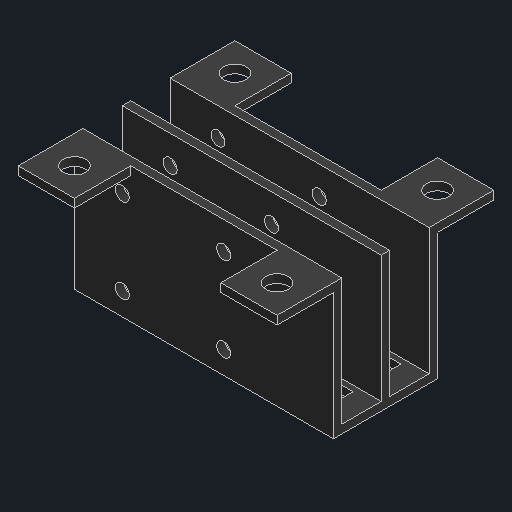
# Autodesk Inventor part: convertor_base
Saved by Autodesk Inventor 2026.1 (Build 301233020, 233B)
## iProperties
Created: 2025-11-26
Part Number: convertor_base
Material: 고무, 검은색
Document SubType Name: Modeling
Designer: jaewook
Density: 0.93 g/cm^3
Appearance: 고무 - 검은색
Author: jaewook
Autodesk Inventor part; units mm, degrees
ref_plane "YZ Plane" through (0, 0, 0) normal (1, 0, 0) x (0, 1, 0)
ref_plane "XZ Plane" through (0, 0, 0) normal (0, 1, 0) x (-1, 0, 0)
ref_plane "XY Plane" through (0, 0, 0) normal (0, 0, 1) x (1, 0, 0)
sketch "스케치1" plane through (0, 0, 0) normal (1, 0, 0) x (0, 1, 0)
  line L0 (12, -9.25) -> (-12, -9.25)
  line L1 (-12, -9.25) -> (-12, 9.25)
  line L2 (-12, 9.25) -> (12, 9.25)
  line L3 (12, 9.25) -> (12, -9.25)
  line L4 (12, -9.25) -> (-12, 9.25) construction
  line L5 (-12, -9.25) -> (12, 9.25) construction
  line L6 (12, 7.75) -> (-10.5, 7.75)
  line L7 (-10.5, 7.75) -> (-10.5, 0.75)
  line L8 (-10.5, 0.75) -> (12, 0.75)
  line L9 (12, 0.75) -> (12, 7.75)
  line L10 (-10.5, -7.75) -> (12, -7.75)
  line L11 (-10.5, -0.75) -> (-10.5, -7.75)
  line L12 (12, -0.75) -> (-10.5, -0.75)
  line L13 (12, 9.25) -> (13.5, 9.25)
  line L14 (13.5, 9.25) -> (13.5, -9.25)
  line L15 (13.5, -9.25) -> (12, -9.25)
  line L16 (12, -9.25) -> (12, 9.25)
  point P0 (0, 0)
  point P1 (12, -7.75)
  point P2 (12, -0.75)
  point P3 (-10, 7.75)
  point P4 (-10, -7.75)
  point P5 (-10, 0.75)
  point P6 (-10, -0.75)
  point P7 (-10, -0.75)
  point P8 (-10, -7.75)
  point P9 (12, 7.75)
  point P10 (12, -7.75)
  dimension "d0" = 24
  dimension "d1" = 18.5
  dimension "d2" = 22.5
  dimension "d3" = 7
  dimension "d4" = 1.5
  dimension "d7" = 8.5
  dimension "d18" = 1.5
  constraints: 34 end point, 6 parallel, 3 horizontal, 3 perpendicular, 2 midpoint, 1 collinear, 1 point on line, 1 vertical, 7 other
  measures "d0" distance of L1.end L2.end
  measures "d1" distance of L0.end L1.end
  measures "d2" distance of L8.end L7.end
  measures "d3" distance of L7.end L6.end
  measures "d4" distance between parallel lines of L2 L6
  measures "d7" distance of L7.end L10.start
  measures "d18" distance of L14.end L15.end
extrude "돌출1" add sketch "스케치1" against normal blind 45 contours L0 L1 L2 L3 L6 L7 L8 L12 L11 L10
sketch "스케치2" plane through (0, 0, 0) normal (1, 0, 0) x (0, 0, -1)
  line L0 (-9.25, -12) -> (9.25, -12) projected
  line L1 (-9.25, 12) -> (-9.25, -12) projected
  line L2 (-9.25, 12) -> (9.25, 12)
  line L3 (9.25, 12) -> (9.25, -12)
  line L4 (9.25, -12) -> (-9.25, -12)
  line L5 (-9.25, -12) -> (-9.25, 12)
  line L6 (9.25, 12) -> (-9.25, 12)
  line L7 (-9.25, 12) -> (-7.75, 12) projected
  point P0 (0, 0)
  constraints: 10 end point, 2 collinear, 2 parallel, 1 horizontal, 1 perpendicular
extrude "돌출2" add sketch "스케치2" along normal blind 1
sketch "스케치4" plane through (-45, -12, 9.25) normal (0, 0, 1) x (1, 0, 0)
  circle A0 centre (8.5, 19) radius 1.25 projected
  circle A1 centre (26.5, 19) radius 1.25 projected
  circle A2 centre (26.5, 4) radius 1.25 projected
  circle A3 centre (8.5, 4) radius 1.25 projected
  point P0 (45, 12)
extrude "돌출3" cut sketch "스케치4" against normal blind 45
sketch "스케치9" plane through (0, 12, 7.75) normal (0, 1, 0) x (1, 0, 0)
  line L0 (-45, 7) -> (-45, 8.5) projected
  line L1 (0, 7) -> (-45, 7) projected
  line L2 (-45, -1.5) -> (1, -1.5) projected
  line L3 (-45, 17) -> (1, 17) projected
  line L4 (-45, 17) -> (-35, 17)
  line L5 (-45, -1.5) -> (-35, -1.5)
  line L6 (-35, -1.5) -> (-35, -11.5)
  line L7 (-35, -11.5) -> (-45, -11.5)
  line L8 (-45, -11.5) -> (-45, -1.5)
  circle A0 centre (-40, -6.5) radius 2
  line L9 (-45, 7.75) -> (0, 7.75) construction
  line L10 (-22, -1.5) -> (-22, 17) construction
  line L11 (-35, 17) -> (-35, 27)
  line L12 (-35, 27) -> (-45, 27)
  line L13 (-45, 27) -> (-45, 17)
  circle A1 centre (-40, 22) radius 2
  line L14 (-45, 17) -> (-35, 17)
  line L15 (1, 17) -> (-9, 17)
  line L16 (1, -1.5) -> (-9, -1.5)
  line L17 (-9, -1.5) -> (-9, -11.5)
  line L18 (-9, -11.5) -> (1, -11.5)
  line L19 (1, -11.5) -> (1, -1.5)
  circle A2 centre (-4, -6.5) radius 2
  circle A3 centre (-4, 22) radius 2
  line L20 (-9, 17) -> (-9, 27)
  line L21 (-9, 27) -> (1, 27)
  line L22 (1, 27) -> (1, 17)
  line L23 (1, 17) -> (-9, 17)
  point P0 (-9, 17)
  dimension "d31" = 10
  dimension "d32" = 10
  dimension "d33" = 4
  dimension "d34" = 5
  dimension "d35" = 5
  constraints: 40 end point, 11 symmetric about line, 4 centre point, 3 midpoint, 3 parallel, 2 horizontal, 2 perpendicular, 3 other
  measures "d31" distance of L6.end L7.end
  measures "d32" distance of L5.end L6.end
  measures "d33" diameter of A0
  measures "d34" distance from line of L7 A0.centre
  measures "d35" distance from line of L6 A0.centre
extrude "돌출6" add sketch "스케치9" against normal blind 1.5
sketch "스케치10" plane through (0, 0, 0) normal (-1, 0, 0) x (0, 0, 1)
  line L0 (-0.75, -10.5) -> (-0.75, 12) projected
  line L1 (-7.75, 12) -> (-0.75, 12) projected
  line L2 (-7.75, 12) -> (-7.75, -10.5) projected
  line L3 (-7.75, -10.5) -> (-0.75, -10.5) projected
  line L4 (1.75, 9.5) -> (1.75, -10.5) projected
  line L5 (1.75, -10.5) -> (7.75, -10.5) projected
  line L6 (7.75, 9.5) -> (7.75, -10.5) projected
  line L7 (1.75, 9.5) -> (7.75, 9.5) projected
  line L8 (0.75, 12) -> (0.75, -10.5) projected
  line L9 (0.75, -10.5) -> (7.75, -10.5) projected
  line L10 (7.75, -10.5) -> (7.75, 12) projected
  line L11 (0.75, 12) -> (7.75, 12) projected
  point P0 (0, 0)
  point P1 (1.75, -10.5)
  point P2 (1.75, 10.75)
  point P3 (7.75, 9.5)
extrude "돌출7" cut sketch "스케치10" against normal blind 10
sketch "스케치11" plane through (-45, -10.5, 7.75) normal (0, 1, 0) x (1, 0, 0)
  line L0 (0, 15.5) -> (46, 15.5) projected
  line L1 (0, 8.5) -> (0, 15.5) projected
  line L2 (46, 15.5) -> (46, 8.5) projected
  line L3 (0, 8.5) -> (0, 7)
  line L4 (46, 8.5) -> (0, 8.5) projected
  line L5 (46, 8.5) -> (46, 7)
  line L6 (0, 7.75) -> (46, 7.75) construction
  line L7 (23, 15.5) -> (23, 8.5) construction
  line L8 (0, 12) -> (46, 12) construction
  line L9 (4, 9.5) -> (42, 9.5)
  line L10 (42, 9.5) -> (42, 14.5)
  line L11 (42, 14.5) -> (4, 14.5)
  line L12 (4, 14.5) -> (4, 9.5)
  line L13 (4, 9.5) -> (42, 14.5) construction
  line L14 (42, 9.5) -> (4, 14.5) construction
  line L15 (4, 6) -> (42, 6)
  line L16 (42, 6) -> (42, 1)
  line L17 (42, 1) -> (4, 1)
  line L18 (4, 1) -> (4, 6)
  line L19 (0, 7.75) -> (46, 7.75) construction
  line L20 (0, 8.5) -> (46, 8.5) projected
  point P0 (45, 7.75)
  point P1 (23, 12)
  dimension "d40" = 1
  dimension "d41" = 4
  constraints: 32 end point, 9 midpoint, 4 symmetric about line, 3 parallel, 2 perpendicular, 1 horizontal, 1 vertical
  measures "d40" distance between parallel lines of L11 L0
  measures "d41" distance between parallel lines of L2 L10
extrude "돌출8" cut sketch "스케치11" against normal blind 10 contours L12 L11 L10 L9 | L15 L16 L17 L18
